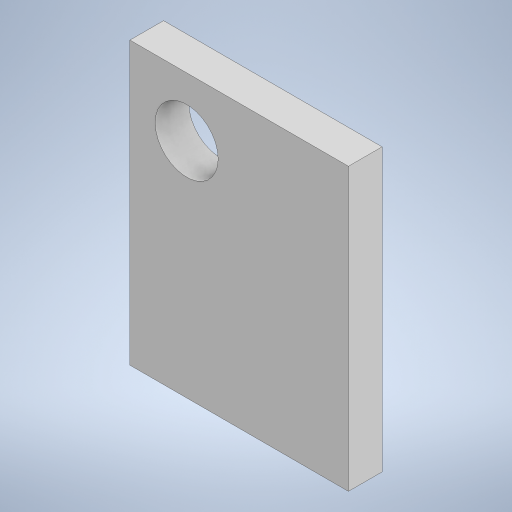
# Autodesk Inventor part: vl53l0x
Saved by Autodesk Inventor 2023 (Build 270158000, 158)
## iProperties
Created: 2024-03-04
Part Number: vl53l0x
Material: Generic
Document SubType Name: Modeling
Designer: pavel
Density: 1 g/cm^3
Appearance: Default
Author: pavel
Autodesk Inventor part; units mm, degrees
ref_plane "YZ Plane" through (0, 0, 0) normal (1, 0, 0) x (0, 1, 0)
ref_plane "XZ Plane" through (0, 0, 0) normal (0, 1, 0) x (-1, 0, 0)
ref_plane "XY Plane" through (0, 0, 0) normal (0, 0, 1) x (1, 0, 0)
sketch "Sketch1" plane through (0, 0, 0) normal (0, 0, 1) x (1, 0, 0)
  line L0 (0, 0) -> (10.4, 0)
  line L1 (10.4, 0) -> (10.4, 13.4)
  line L2 (10.4, 13.4) -> (0, 13.4)
  line L3 (0, 13.4) -> (0, 0)
  dimension "d0" = 10.4
  dimension "d1" = 13.4
  constraints: 8 end point, 2 parallel, 1 horizontal, 1 perpendicular
  measures "d0" distance of L2.end L1.end
  measures "d1" distance of L1.end L0.end
extrude "Extrusion1" add sketch "Sketch1" along normal blind 1.6
sketch "Sketch2" plane through (0, 0, 1.6) normal (0, 0, 1) x (1, 0, 0)
  line L0 (10.4, 13.4) -> (0, 13.4) projected
  line L1 (0, 13.4) -> (0, 0) projected
  point P0 (2.7, 10.6)
  dimension "d4" = 2.8
  dimension "d5" = 2.7
  measures "d4" distance from line of L0 point (2.7, 10.6)
  measures "d5" distance from line of L1 point (2.7, 10.6)
hole "Hole1" at (2.7, 10.6, 1.6) direction (0, 0, -1) diameter 3 depth 1.6
body "Solid1"
